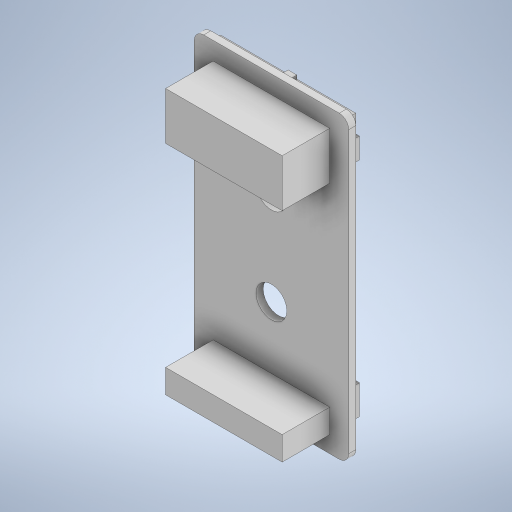
# Autodesk Inventor part: нижняя часть блока аккумов
Saved by Autodesk Inventor 2023.1 (Build 271208000, 208)
## iProperties
Created: 2023-03-03
Part Number: нижняя часть блока аккумов
Material: Типовые
Document SubType Name: Modeling
Designer: User
Density: 1 g/cm^3
Appearance: По умолчанию
Author: User
Autodesk Inventor part; units mm, degrees
ref_plane "YZ Plane" through (0, 0, 0) normal (1, 0, 0) x (0, 1, 0)
ref_plane "XZ Plane" through (0, 0, 0) normal (0, 1, 0) x (-1, 0, 0)
ref_plane "XY Plane" through (0, 0, 0) normal (0, 0, 1) x (1, 0, 0)
sketch "Эскиз1" plane through (0, 0, 0) normal (0, 0, 1) x (1, 0, 0)
  line L0 (-14.25, 29.75) -> (14.25, 29.75)
  line L1 (14.25, 29.75) -> (14.25, -29.75)
  line L2 (14.25, -29.75) -> (-14.25, -29.75)
  line L3 (-14.25, -29.75) -> (-14.25, 29.75)
  line L4 (0, -41.65) -> (0, 41.65) projected
  line L5 (-19.95, 0) -> (19.95, 0) projected
  line L6 (-12.25, 27.75) -> (12.25, 27.75)
  line L7 (12.25, 27.75) -> (12.25, -27.75)
  line L8 (12.25, -27.75) -> (-12.25, -27.75)
  line L9 (-12.25, -27.75) -> (-12.25, 27.75)
  point P0 (0, 0)
  dimension "d0" = 28.5
  dimension "d1" = 59.5
  dimension "d2" = 2
  constraints: 16 end point, 4 parallel, 2 perpendicular, 1 horizontal, 5 other
  measures "d0" distance between parallel lines of L1 L3
  measures "d1" distance between parallel lines of L2 L0
  measures "d2" distance between parallel lines of L3 L9
extrude "Выдавливание1" add sketch "Эскиз1" along normal blind 2 contours L0 L4 L6 L9 L5 L3 | L0 L1 L5 L7 L6 L4 | L5 L9 L8 L4 L2 L3 | L1 L2 L4 L8 L7 L5
sketch "Эскиз2" plane through (0, 0, 2) normal (0, 0, 1) x (1, 0, 0)
  line L0 (-16.25, 31.5) -> (16.25, 31.5)
  line L1 (16.25, 31.5) -> (16.25, -31.5)
  line L2 (16.25, -31.5) -> (-16.25, -31.5)
  line L3 (-16.25, -31.5) -> (-16.25, 31.5)
  line L4 (0, -44.1) -> (0, 44.1) projected
  line L5 (-22.75, 0) -> (22.75, 0) projected
  point P0 (0, 0)
  dimension "d5" = 63
  dimension "d6" = 32.5
  constraints: 8 end point, 2 parallel, 1 horizontal, 1 perpendicular, 2 other
  measures "d5" distance between parallel lines of L2 L0
  measures "d6" distance between parallel lines of L1 L3
extrude "Выдавливание2" add sketch "Эскиз2" along normal blind 1.5
sketch "Эскиз3" plane through (0, 0, 2) normal (0, 0, -1) x (-1, 0, 0)
  line L0 (15, -30.5) -> (-15, -30.5)
  line L1 (-15, -30.5) -> (-15, 30.5)
  line L2 (-15, 30.5) -> (15, 30.5)
  line L3 (15, 30.5) -> (15, -30.5)
  line L4 (0, -44.1) -> (0, 44.1) projected
  line L5 (22.75, 0) -> (-22.75, 0) projected
  line L6 (14.25, -29.75) -> (-14.25, -29.75) projected
  line L7 (1.6881, -30.5) -> (-1.7436, -30.5)
  line L8 (-1.7436, -30.5) -> (-1.7436, -29.75)
  line L9 (-1.7436, -29.75) -> (1.6881, -29.75)
  line L10 (1.6881, -29.75) -> (1.6881, -30.5)
  line L11 (1.6881, 29.75) -> (-1.8544, 29.75)
  line L12 (-1.8544, 29.75) -> (-1.8544, 30.5)
  line L13 (-1.8544, 30.5) -> (1.6881, 30.5)
  line L14 (1.6881, 30.5) -> (1.6881, 29.75)
  line L15 (14.25, 29.75) -> (14.25, -29.75) projected
  line L16 (15, 22.8864) -> (14.25, 22.8864)
  line L17 (14.25, 22.8864) -> (14.25, 25.9613)
  line L18 (14.25, 25.9613) -> (15, 25.9613)
  line L19 (15, 25.9613) -> (15, 22.8864)
  line L20 (15, -24.3425) -> (14.25, -24.3425)
  line L21 (14.25, -24.3425) -> (14.25, -20.2031)
  line L22 (14.25, -20.2031) -> (15, -20.2031)
  line L23 (15, -20.2031) -> (15, -24.3425)
  line L24 (-14.2166, -25.1255) -> (-15, -25.1255)
  line L25 (-15, -25.1255) -> (-15, -18.943)
  line L26 (-15, -18.943) -> (-14.2166, -18.943)
  line L27 (-14.2166, -18.943) -> (-14.2166, -25.1255)
  line L28 (-14.2166, 21.6162) -> (-15, 21.6162)
  line L29 (-15, 21.6162) -> (-15, 25.9613)
  line L30 (-15, 25.9613) -> (-14.2166, 25.9613)
  line L31 (-14.2166, 25.9613) -> (-14.2166, 21.6162)
  point P0 (0, 0)
  point P1 (0, 29.75)
  point P2 (0, 30.5)
  point P3 (1.6881, -29.75)
  dimension "d9" = 61
  dimension "d10" = 30
  constraints: 56 end point, 14 parallel, 10 point on line, 7 horizontal, 7 perpendicular, 2 other
  measures "d9" distance between parallel lines of L2 L0
  measures "d10" distance between parallel lines of L3 L1
extrude "Выдавливание3" add sketch "Эскиз3" along normal blind 2 contours L0 L4 L6 L10 | L20 L15 L22 L3 | L0 L8 L6 L4 | L16 L15 L18 L3 | L1 L26 L27 L24 | L11 L12 L2 L4 | L1 L30 L31 L28
sketch "Эскиз4" plane through (0, 0, 3.5) normal (0, 0, 1) x (1, 0, 0)
  circle A0 centre (0, -10) radius 3.25
  circle A1 centre (0, 10) radius 3.25
  line L0 (-22.75, 0) -> (22.75, 0) projected
  point P0 (0, 0)
  dimension "d13" = 6.5
  dimension "d14" = 6.5
  dimension "d15" = 20
  constraints: 2 centre point, 1 symmetric about line
  measures "d13" diameter of A0
  measures "d14" diameter of A1
  measures "d15" distance of A1.centre A0.centre
extrude "Выдавливание4" cut sketch "Эскиз4" against normal blind 2
fillet "Сопряжение1" radius 2 4 edges at (-16.25, 31.5, 2.75) (16.25, 31.5, 2.75) (16.25, -31.5, 2.75) (-16.25, -31.5, 2.75)
sketch "Эскиз5" plane through (0, 0, 3.5) normal (0, 0, 1) x (1, 0, 0)
  line L0 (-12.25, 27.75) -> (12.25, 27.75) projected
  line L1 (12.25, 27.75) -> (12.25, -27.75) projected
  line L2 (-12.25, 27.75) -> (12.25, 27.75)
  line L3 (12.25, 27.75) -> (12.25, 17.75)
  line L4 (12.25, 17.75) -> (-12.25, 17.75)
  line L5 (-12.25, 17.75) -> (-12.25, 27.75)
  line L6 (-12.25, -27.75) -> (-12.25, 27.75) projected
  line L7 (12.25, -28.0211) -> (-12.25, -28.0211)
  line L8 (-12.25, -28.0211) -> (-12.25, -23.0211)
  line L9 (-12.25, -23.0211) -> (12.25, -23.0211)
  line L10 (12.25, -23.0211) -> (12.25, -28.0211)
  point P0 (0, 0)
  point P1 (12.25, -23.0211)
  dimension "d19" = 10
  dimension "d20" = 5
  constraints: 16 end point, 4 parallel, 3 point on line, 2 horizontal, 2 perpendicular
  measures "d19" distance between parallel lines of L0 L4
  measures "d20" distance between parallel lines of L9 L7
extrude "Выдавливание5" add sketch "Эскиз5" along normal blind 10 contours L0 L1 L4 L5 | L9 L1 L10 L7 L8 L6
